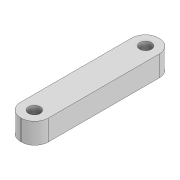
# Autodesk Inventor part: Hand4
Saved by Autodesk Inventor 2022 (Build 260153000, 153)
## iProperties
Created: 2021-06-21
Part Number: Hand4
Material: Generic
Document SubType Name: Modeling
Designer: Prajwal Patil
Density: 1 g/cm^3
Appearance: Default
Author: Prajwal Patil
Autodesk Inventor part; units mm, degrees
ref_plane "YZ Plane" through (0, 0, 0) normal (1, 0, 0) x (0, 1, 0)
ref_plane "XZ Plane" through (0, 0, 0) normal (0, 1, 0) x (-1, 0, 0)
ref_plane "XY Plane" through (0, 0, 0) normal (0, 0, 1) x (1, 0, 0)
sketch "Sketch1" plane through (0, 0, 0) normal (0, 1, 0) x (-1, 0, 0)
  line L0 (9.8538, 29.2055) -> (-0.3062, 29.2055)
  line L1 (-0.3062, 29.2055) -> (-0.3062, -21.5945)
  line L2 (-0.3062, -21.5945) -> (9.8538, -21.5945)
  line L3 (9.8538, -21.5945) -> (9.8538, 29.2055)
  line L4 (4.7738, -21.5945) -> (4.7738, -16.6415)
  line L5 (4.7738, 29.2055) -> (4.7738, 24.2525)
  circle A0 centre (4.7738, 24.2525) radius 2.159
  circle A1 centre (4.7738, -16.6415) radius 2.159
  point P0 (0, 0)
  dimension "d0" = 10.16
  dimension "d1" = 50.8
  dimension "d2" = 4.953
  dimension "d3" = 4.953
  dimension "d4" = 4.318
  dimension "d5" = 4.318
  constraints: 12 end point, 2 centre point, 2 coincident, 2 midpoint, 2 parallel, 2 vertical, 1 horizontal, 1 perpendicular
  measures "d0" distance of L2.end L1.end
  measures "d1" distance of L1.end L0.end
  measures "d2" distance of L4.start L4.end
  measures "d3" distance of L5.start L5.end
  measures "d4" diameter of A0
  measures "d5" diameter of A1
extrude "Extrusion1" add sketch "Sketch1" along normal blind 7.62
fillet "Fillet1" radius 4.953 1 edges at (0.3062, 3.81, -21.5945)
fillet "Fillet2" radius 4.953 3 edges at (-9.8538, 3.81, -21.5945) (0.3062, 3.81, 29.2055) (-9.8538, 3.81, 29.2055)
body "Solid1"
